Autodesk Fusion 360 part; units mm, degrees
note: some values were not read from the file. Chosen so that the rebuilt part matches the saved one: which face or edge a step refers to. Set by a fixed rule: which sketch regions a step uses.
(part 2 of 2)
  spline S262 degree 3 poles (19.3379, -14.9324) (18.8966, -14.9324) (18.4636, -14.9324) (18.0258, -14.9324) knots 0 0 0 0 1 1 1 1
  spline S263 degree 3 poles (18.0258, -14.9324) (18.0258, -13.8885) (18.0258, -12.8484) (18.0258, -11.8015) knots 0 0 0 0 1 1 1 1
  spline S264 degree 3 poles (18.0258, -11.8015) (18.3648, -11.8015) (18.7049, -11.8015) (19.0516, -11.8015) knots 0 0 0 0 1 1 1 1
  spline S265 degree 3 poles (19.0516, -11.8015) (19.0516, -10.138) (19.0516, -8.4811) (19.0516, -6.8195) knots 0 0 0 0 1 1 1 1
  spline S266 degree 3 poles (19.0516, -6.8195) (19.5983, -6.8195) (20.1384, -6.8195) (20.6851, -6.8195) knots 0 0 0 0 1 1 1 1
  spline S267 degree 3 poles (20.6851, -6.8195) (20.6851, -8.4753) (20.6851, -10.1322) (20.6851, -11.7957) knots 0 0 0 0 1 1 1 1
  spline S268 degree 3 poles (20.6851, -11.7957) (21.0317, -11.7957) (21.3719, -11.7957) (21.7168, -11.7957) knots 0 0 0 0 1 1 1 1
  spline S269 degree 3 poles (21.7168, -11.7957) (21.7168, -12.8425) (21.7168, -13.8827) (21.7168, -14.9324) knots 0 0 0 0 1 1 1 1
  spline S270 degree 3 poles (21.7168, -14.9324) (20.9273, -14.9324) (20.1368, -14.9324) (19.3379, -14.9324) knots 0 0 0 0 1 1 1 1
  spline S271 degree 3 poles (16.0875, -14.9324) (15.3573, -14.9324) (14.6354, -14.9324) (13.9087, -14.9324) knots 0 0 0 0 1 1 1 1
  spline S272 degree 3 poles (13.9087, -14.9324) (13.9087, -13.8886) (13.9087, -12.8484) (13.9087, -11.8016) knots 0 0 0 0 1 1 1 1
  spline S273 degree 3 poles (13.9087, -11.8016) (14.2476, -11.8016) (14.5877, -11.8016) (14.9344, -11.8016) knots 0 0 0 0 1 1 1 1
  spline S274 degree 3 poles (14.9344, -11.8016) (14.9344, -10.1381) (14.9344, -8.4812) (14.9344, -6.8195) knots 0 0 0 0 1 1 1 1
  spline S275 degree 3 poles (14.9344, -6.8195) (15.4811, -6.8195) (16.0212, -6.8195) (16.5679, -6.8195) knots 0 0 0 0 1 1 1 1
  spline S276 degree 3 poles (16.5679, -6.8195) (16.5679, -8.4752) (16.5679, -10.1321) (16.5679, -11.7956) knots 0 0 0 0 1 1 1 1
  spline S277 degree 3 poles (16.5679, -11.7956) (16.9145, -11.7956) (17.2547, -11.7956) (17.5996, -11.7956) knots 0 0 0 0 1 1 1 1
  spline S278 degree 3 poles (17.5996, -11.7956) (17.5996, -12.8425) (17.5996, -13.8826) (17.5996, -14.9324) knots 0 0 0 0 1 1 1 1
  spline S279 degree 3 poles (17.5996, -14.9324) (17.0991, -14.9324) (16.5975, -14.9324) (16.0875, -14.9324) knots 0 0 0 0 1 1 1 1
  spline S280 degree 3 poles (5.2528, -14.5323) (5.2528, -14.6681) (5.2528, -14.7955) (5.2528, -14.9276) knots 0 0 0 0 1 1 1 1
  spline S281 degree 3 poles (5.2528, -14.9276) (4.02, -14.9276) (2.7909, -14.9276) (1.5571, -14.9276) knots 0 0 0 0 1 1 1 1
  spline S282 degree 3 poles (1.5571, -14.9276) (1.5571, -13.8885) (1.5571, -12.8484) (1.5571, -11.8015) knots 0 0 0 0 1 1 1 1
  spline S283 degree 3 poles (1.5571, -11.8015) (1.8961, -11.8015) (2.2362, -11.8015) (2.5829, -11.8015) knots 0 0 0 0 1 1 1 1
  spline S284 degree 3 poles (2.5829, -11.8015) (2.5829, -10.138) (2.5829, -8.4811) (2.5829, -6.8195) knots 0 0 0 0 1 1 1 1
  spline S285 degree 3 poles (2.5829, -6.8195) (3.1296, -6.8195) (3.6697, -6.8195) (4.2164, -6.8195) knots 0 0 0 0 1 1 1 1
  spline S286 degree 3 poles (4.2164, -6.8195) (4.2164, -8.4753) (4.2164, -10.1322) (4.2164, -11.7957) knots 0 0 0 0 1 1 1 1
  spline S287 degree 3 poles (4.2164, -11.7957) (4.563, -11.7957) (4.9032, -11.7957) (5.2528, -11.7957) knots 0 0 0 0 1 1 1 1
  spline S288 degree 3 poles (5.2528, -11.7957) (5.2528, -12.7095) (5.2528, -13.6168) (5.2528, -14.5323) knots 0 0 0 0 1 1 1 1
  spline S289 degree 3 poles (19.0545, 0.9863) (19.0545, 1.7388) (19.0545, 2.4829) (19.0545, 3.2336) knots 0 0 0 0 1 1 1 1
  spline S290 degree 3 poles (19.0545, 3.2336) (18.7109, 3.2336) (18.3707, 3.2336) (18.0258, 3.2336) knots 0 0 0 0 1 1 1 1
  spline S291 degree 3 poles (18.0258, 3.2336) (18.0258, 4.2805) (18.0258, 5.3206) (18.0258, 6.3655) knots 0 0 0 0 1 1 1 1
  spline S292 degree 3 poles (18.0258, 6.3655) (19.2538, 6.3655) (20.4829, 6.3655) (21.7167, 6.3655) knots 0 0 0 0 1 1 1 1
  spline S293 degree 3 poles (21.7167, 6.3655) (21.7167, 5.3265) (21.7167, 4.2863) (21.7167, 3.2395) knots 0 0 0 0 1 1 1 1
  spline S294 degree 3 poles (21.7167, 3.2395) (21.3778, 3.2395) (21.0376, 3.2395) (20.6909, 3.2395) knots 0 0 0 0 1 1 1 1
  spline S295 degree 3 poles (20.6909, 3.2395) (20.6909, 1.576) (20.6909, -0.0809) (20.6909, -1.7426) knots 0 0 0 0 1 1 1 1
  spline S296 degree 3 poles (20.6909, -1.7426) (20.1443, -1.7426) (19.6042, -1.7426) (19.0545, -1.7426) knots 0 0 0 0 1 1 1 1
  spline S297 degree 3 poles (19.0545, -1.7426) (19.0545, -0.8365) (19.0545, 0.0708) (19.0545, 0.9863) knots 0 0 0 0 1 1 1 1
  spline S298 degree 3 poles (16.5709, -0.0972) (16.5709, -0.6496) (16.5709, -1.1937) (16.5709, -1.7426) knots 0 0 0 0 1 1 1 1
  spline S299 degree 3 poles (16.5709, -1.7426) (16.0271, -1.7426) (15.487, -1.7426) (14.9403, -1.7426) knots 0 0 0 0 1 1 1 1
  spline S300 degree 3 poles (14.9403, -1.7426) (14.9403, -0.0868) (14.9403, 1.5701) (14.9403, 3.2336) knots 0 0 0 0 1 1 1 1
  spline S301 degree 3 poles (14.9403, 3.2336) (14.5937, 3.2336) (14.2535, 3.2336) (13.9086, 3.2336) knots 0 0 0 0 1 1 1 1
  spline S302 degree 3 poles (13.9086, 3.2336) (13.9086, 4.2805) (13.9086, 5.3206) (13.9086, 6.3655) knots 0 0 0 0 1 1 1 1
  spline S303 degree 3 poles (13.9086, 6.3655) (15.1366, 6.3655) (16.3657, 6.3655) (17.5996, 6.3655) knots 0 0 0 0 1 1 1 1
  spline S304 degree 3 poles (17.5996, 6.3655) (17.5996, 5.3265) (17.5996, 4.2863) (17.5996, 3.2395) knots 0 0 0 0 1 1 1 1
  spline S305 degree 3 poles (17.5996, 3.2395) (17.2606, 3.2395) (16.9204, 3.2395) (16.5709, 3.2395) knots 0 0 0 0 1 1 1 1
  spline S306 degree 3 poles (16.5709, 3.2395) (16.5709, 2.1256) (16.5709, 1.0184) (16.5709, -0.0972) knots 0 0 0 0 1 1 1 1
  spline S307 degree 3 poles (19.8763, -5.7028) (19.5057, -6.0811) (19.0512, -6.2863) (18.5382, -6.3084) knots 0 0 0 0 1 1 1 1
  spline S308 degree 3 poles (18.5382, -6.3084) (17.8871, -6.3365) (17.2339, -6.3152) (16.5762, -6.3152) knots 0 0 0 0 1 1 1 1
  spline S309 degree 3 poles (16.5762, -6.3152) (16.5762, -4.9588) (16.5762, -3.5911) (16.5762, -2.2154) knots 0 0 0 0 1 1 1 1
  spline S310 degree 3 poles (16.5762, -2.2154) (16.5981, -2.2154) (16.6194, -2.2154) (16.6407, -2.2154) knots 0 0 0 0 1 1 1 1
  spline S311 degree 3 poles (16.6407, -2.2154) (17.1769, -2.2154) (17.713, -2.2138) (18.2492, -2.216) knots 0 0 0 0 1 1 1 1
  spline S312 degree 3 poles (18.2492, -2.216) (18.6308, -2.2175) (19.0001, -2.2829) (19.3445, -2.4547) knots 0 0 0 0 1 1 1 1
  spline S313 degree 3 poles (19.3445, -2.4547) (19.8492, -2.7066) (20.1823, -3.104) (20.3251, -3.6506) knots 0 0 0 0 1 1 1 1
  spline S314 degree 3 poles (20.3251, -3.6506) (20.4718, -4.2122) (20.439, -4.763) (20.1704, -5.2845) knots 0 0 0 0 1 1 1 1
  spline S315 degree 3 poles (20.1704, -5.2845) (20.0939, -5.4329) (19.9781, -5.561) (19.8763, -5.7028) knots 0 0 0 0 1 1 1 1
  spline S316 degree 3 poles (18.5377, -5.3752) (18.927, -5.274) (19.1788, -5.0271) (19.3006, -4.6473) knots 0 0 0 0 1 1 1 1
  spline S317 degree 3 poles (19.3006, -4.6473) (19.3662, -4.443) (19.3674, -4.2332) (19.3366, -4.0219) knots 0 0 0 0 1 1 1 1
  spline S318 degree 3 poles (19.3366, -4.0219) (19.265, -3.5312) (18.898, -3.1807) (18.4023, -3.1496) knots 0 0 0 0 1 1 1 1
  spline S319 degree 3 poles (18.4023, -3.1496) (18.1424, -3.1333) (17.881, -3.1411) (17.6203, -3.1384) knots 0 0 0 0 1 1 1 1
  spline S320 degree 3 poles (17.6203, -3.1384) (17.6161, -3.1384) (17.6118, -3.1449) (17.6084, -3.1476) knots 0 0 0 0 1 1 1 1
  spline S321 degree 3 poles (17.6084, -3.1476) (17.6084, -3.8994) (17.6084, -4.6506) (17.6084, -5.4225) knots 0 0 0 0 1 1 1 1
  spline S322 degree 3 poles (17.6084, -5.4225) (17.9168, -5.4076) (18.2205, -5.3929) (18.5377, -5.3752) knots 0 0 0 0 1 1 1 1
  spline S323 degree 3 poles (15.3406, -2.4936) (16.0423, -3.0161) (16.0475, -4.4321) (15.0414, -4.8191) knots 0 0 0 0 1 1 1 1
  spline S324 degree 3 poles (15.0414, -4.8191) (15.3108, -5.3205) (15.5798, -5.8213) (15.8523, -6.3286) knots 0 0 0 0 1 1 1 1
  spline S325 degree 3 poles (15.8523, -6.3286) (15.4534, -6.3286) (15.0653, -6.3286) (14.675, -6.3286) knots 0 0 0 0 1 1 1 1
  spline S326 degree 3 poles (14.675, -6.3286) (14.4647, -5.8864) (14.2534, -5.4444) (14.0449, -5.001) knots 0 0 0 0 1 1 1 1
  spline S327 degree 3 poles (14.0449, -5.001) (14.0209, -4.95) (13.9954, -4.9272) (13.9354, -4.9294) knots 0 0 0 0 1 1 1 1
  spline S328 degree 3 poles (13.9354, -4.9294) (13.7889, -4.9347) (13.6421, -4.9311) (13.4889, -4.9311) knots 0 0 0 0 1 1 1 1
  spline S329 degree 3 poles (13.4889, -4.9311) (13.4889, -5.3983) (13.4889, -5.8607) (13.4889, -6.3271) knots 0 0 0 0 1 1 1 1
  spline S330 degree 3 poles (13.4889, -6.3271) (13.1422, -6.3271) (12.8021, -6.3271) (12.4579, -6.3271) knots 0 0 0 0 1 1 1 1
  spline S331 degree 3 poles (12.4579, -6.3271) (12.4579, -4.9586) (12.4579, -3.5907) (12.4579, -2.2171) knots 0 0 0 0 1 1 1 1
  spline S332 degree 3 poles (12.4579, -2.2171) (12.479, -2.2161) (12.5003, -2.2142) (12.5215, -2.2142) knots 0 0 0 0 1 1 1 1
  spline S333 degree 3 poles (12.5215, -2.2142) (13.1604, -2.2141) (13.7992, -2.2129) (14.4381, -2.2146) knots 0 0 0 0 1 1 1 1
  spline S334 degree 3 poles (14.4381, -2.2146) (14.7645, -2.2155) (15.0702, -2.2889) (15.3406, -2.4936) knots 0 0 0 0 1 1 1 1
  spline S335 degree 3 poles (14.5491, -3.9706) (14.7482, -3.8541) (14.8308, -3.6559) (14.7702, -3.44) knots 0 0 0 0 1 1 1 1
  spline S336 degree 3 poles (14.7702, -3.44) (14.7198, -3.2602) (14.5592, -3.1252) (14.3613, -3.1158) knots 0 0 0 0 1 1 1 1
  spline S337 degree 3 poles (14.3613, -3.1158) (14.1508, -3.1058) (13.9397, -3.1102) (13.7288, -3.1087) knots 0 0 0 0 1 1 1 1
  spline S338 degree 3 poles (13.7288, -3.1087) (13.6496, -3.1082) (13.5705, -3.1087) (13.4928, -3.1087) knots 0 0 0 0 1 1 1 1
  spline S339 degree 3 poles (13.4928, -3.1087) (13.4928, -3.4221) (13.4928, -3.7256) (13.4928, -4.031) knots 0 0 0 0 1 1 1 1
  spline S340 degree 3 poles (13.4928, -4.031) (13.7592, -4.031) (14.02, -4.0354) (14.2806, -4.0285) knots 0 0 0 0 1 1 1 1
  spline S341 degree 3 poles (14.2806, -4.0285) (14.3669, -4.0263) (14.4525, -3.9952) (14.5491, -3.9706) knots 0 0 0 0 1 1 1 1
  spline S342 degree 3 poles (8.8148, -6.2867) (7.9838, -5.9726) (7.5385, -5.3685) (7.4511, -4.4994) knots 0 0 0 0 1 1 1 1
  spline S343 degree 3 poles (7.4511, -4.4994) (7.3936, -3.9287) (7.5204, -3.3995) (7.8763, -2.9414) knots 0 0 0 0 1 1 1 1
  spline S344 degree 3 poles (7.8763, -2.9414) (8.2477, -2.4633) (8.7507, -2.2206) (9.3469, -2.1623) knots 0 0 0 0 1 1 1 1
  spline S345 degree 3 poles (9.3469, -2.1623) (9.8261, -2.1155) (10.2832, -2.1946) (10.7025, -2.4367) knots 0 0 0 0 1 1 1 1
  spline S346 degree 3 poles (10.7025, -2.4367) (11.2593, -2.7583) (11.5798, -3.2502) (11.6844, -3.8784) knots 0 0 0 0 1 1 1 1
  spline S347 degree 3 poles (11.6844, -3.8784) (11.7777, -4.4385) (11.6991, -4.975) (11.3926, -5.4625) knots 0 0 0 0 1 1 1 1
  spline S348 degree 3 poles (11.3926, -5.4625) (11.0607, -5.9903) (10.5708, -6.2819) (9.9625, -6.3817) knots 0 0 0 0 1 1 1 1
  spline S349 degree 3 poles (9.9625, -6.3817) (9.5752, -6.4451) (9.1938, -6.4143) (8.8148, -6.2867) knots 0 0 0 0 1 1 1 1
  spline S350 degree 3 poles (9.7451, -5.4646) (10.0197, -5.4283) (10.2464, -5.3025) (10.4124, -5.0825) knots 0 0 0 0 1 1 1 1
  spline S351 degree 3 poles (10.4124, -5.0825) (10.6866, -4.7192) (10.7297, -4.3093) (10.616, -3.881) knots 0 0 0 0 1 1 1 1
  spline S352 degree 3 poles (10.616, -3.881) (10.4922, -3.415) (10.1205, -3.1151) (9.652, -3.0849) knots 0 0 0 0 1 1 1 1
  spline S353 degree 3 poles (9.652, -3.0849) (9.1837, -3.0546) (8.7796, -3.2983) (8.5947, -3.7278) knots 0 0 0 0 1 1 1 1
  spline S354 degree 3 poles (8.5947, -3.7278) (8.4712, -4.015) (8.4548, -4.3139) (8.5232, -4.6165) knots 0 0 0 0 1 1 1 1
  spline S355 degree 3 poles (8.5232, -4.6165) (8.6538, -5.1952) (9.1669, -5.5546) (9.7451, -5.4646) knots 0 0 0 0 1 1 1 1
  spline S356 degree 3 poles (4.7861, -3.7476) (5.0496, -3.7476) (5.3047, -3.7476) (5.5663, -3.7476) knots 0 0 0 0 1 1 1 1
  spline S357 degree 3 poles (5.5663, -3.7476) (5.5663, -3.2374) (5.5663, -2.7307) (5.5663, -2.219) knots 0 0 0 0 1 1 1 1
  spline S358 degree 3 poles (5.5663, -2.219) (5.9128, -2.219) (6.2529, -2.219) (6.598, -2.219) knots 0 0 0 0 1 1 1 1
  spline S359 degree 3 poles (6.598, -2.219) (6.598, -3.5851) (6.598, -4.9528) (6.598, -6.3259) knots 0 0 0 0 1 1 1 1
  spline S360 degree 3 poles (6.598, -6.3259) (6.2605, -6.3259) (5.9205, -6.3259) (5.5715, -6.3259) knots 0 0 0 0 1 1 1 1
  spline S361 degree 3 poles (5.5715, -6.3259) (5.5715, -5.7784) (5.5715, -5.2277) (5.5715, -4.6731) knots 0 0 0 0 1 1 1 1
  spline S362 degree 3 poles (5.5715, -4.6731) (5.0171, -4.6731) (4.4716, -4.6731) (3.9202, -4.6731) knots 0 0 0 0 1 1 1 1
  spline S363 degree 3 poles (3.9202, -4.6731) (3.9202, -5.2257) (3.9202, -5.7744) (3.9202, -6.3272) knots 0 0 0 0 1 1 1 1
  spline S364 degree 3 poles (3.9202, -6.3272) (3.5742, -6.3272) (3.2342, -6.3272) (2.89, -6.3272) knots 0 0 0 0 1 1 1 1
  spline S365 degree 3 poles (2.89, -6.3272) (2.89, -4.9586) (2.89, -3.5909) (2.89, -2.2187) knots 0 0 0 0 1 1 1 1
  spline S366 degree 3 poles (2.89, -2.2187) (3.23, -2.2187) (3.57, -2.2187) (3.9166, -2.2187) knots 0 0 0 0 1 1 1 1
  spline S367 degree 3 poles (3.9166, -2.2187) (3.9166, -2.7248) (3.9166, -3.2315) (3.9166, -3.7476) knots 0 0 0 0 1 1 1 1
  spline S368 degree 3 poles (3.9166, -3.7476) (4.2079, -3.7476) (4.4928, -3.7476) (4.7861, -3.7476) knots 0 0 0 0 1 1 1 1
  spline S369 degree 3 poles (22.9175, -6.4111) (22.3762, -6.4254) (21.8629, -6.3473) (21.4008, -6.0606) knots 0 0 0 0 1 1 1 1
  spline S370 degree 3 poles (21.4008, -6.0606) (21.263, -5.9751) (21.1384, -5.8684) (21.0063, -5.7703) knots 0 0 0 0 1 1 1 1
  spline S371 degree 3 poles (21.0063, -5.7703) (21.1969, -5.4911) (21.3764, -5.2281) (21.5574, -4.9629) knots 0 0 0 0 1 1 1 1
  spline S372 degree 3 poles (21.5574, -4.9629) (21.8467, -5.2515) (22.1842, -5.4301) (22.5817, -5.489) knots 0 0 0 0 1 1 1 1
  spline S373 degree 3 poles (22.5817, -5.489) (22.7472, -5.5135) (22.9146, -5.5251) (23.0774, -5.4773) knots 0 0 0 0 1 1 1 1
  spline S374 degree 3 poles (23.0774, -5.4773) (23.1505, -5.4558) (23.2248, -5.4235) (23.2856, -5.3785) knots 0 0 0 0 1 1 1 1
  spline S375 degree 3 poles (23.2856, -5.3785) (23.4555, -5.2526) (23.4475, -5.0356) (23.2715, -4.9181) knots 0 0 0 0 1 1 1 1
  spline S376 degree 3 poles (23.2715, -4.9181) (23.1088, -4.8095) (22.9173, -4.7803) (22.7327, -4.7317) knots 0 0 0 0 1 1 1 1
  spline S377 degree 3 poles (22.7327, -4.7317) (22.4467, -4.6562) (22.1557, -4.5935) (21.8784, -4.4933) knots 0 0 0 0 1 1 1 1
  spline S378 degree 3 poles (21.8784, -4.4933) (21.5626, -4.3793) (21.3157, -4.1722) (21.2023, -3.8388) knots 0 0 0 0 1 1 1 1
  spline S379 degree 3 poles (21.2023, -3.8388) (20.9904, -3.2162) (21.2975, -2.5667) (21.9309, -2.2991) knots 0 0 0 0 1 1 1 1
  spline S380 degree 3 poles (21.9309, -2.2991) (22.2119, -2.1804) (22.5074, -2.14) (22.8099, -2.1493) knots 0 0 0 0 1 1 1 1
  spline S381 degree 3 poles (22.8099, -2.1493) (23.3266, -2.1652) (23.8053, -2.3004) (24.2246, -2.6141) knots 0 0 0 0 1 1 1 1
  spline S382 degree 3 poles (24.2246, -2.6141) (24.269, -2.6472) (24.3112, -2.6833) (24.3582, -2.7211) knots 0 0 0 0 1 1 1 1
  spline S383 degree 3 poles (24.3582, -2.7211) (24.1702, -2.9751) (23.9841, -3.2265) (23.7958, -3.481) knots 0 0 0 0 1 1 1 1
  spline S384 degree 3 poles (23.7958, -3.481) (23.5573, -3.2871) (23.2915, -3.1547) (22.9932, -3.0916) knots 0 0 0 0 1 1 1 1
  spline S385 degree 3 poles (22.9932, -3.0916) (22.81, -3.0529) (22.6254, -3.0318) (22.4411, -3.0831) knots 0 0 0 0 1 1 1 1
  spline S386 degree 3 poles (22.4411, -3.0831) (22.3965, -3.0955) (22.3516, -3.1151) (22.3135, -3.1412) knots 0 0 0 0 1 1 1 1
  spline S387 degree 3 poles (22.3135, -3.1412) (22.1419, -3.2588) (22.1442, -3.5034) (22.3312, -3.5903) knots 0 0 0 0 1 1 1 1
  spline S388 degree 3 poles (22.3312, -3.5903) (22.4872, -3.6628) (22.6594, -3.7048) (22.8281, -3.7446) knots 0 0 0 0 1 1 1 1
  spline S389 degree 3 poles (22.8281, -3.7446) (23.1543, -3.8216) (23.4844, -3.8837) (23.789, -4.0313) knots 0 0 0 0 1 1 1 1
  spline S390 degree 3 poles (23.789, -4.0313) (24.0819, -4.1733) (24.316, -4.3737) (24.4065, -4.7003) knots 0 0 0 0 1 1 1 1
  spline S391 degree 3 poles (24.4065, -4.7003) (24.5516, -5.2235) (24.4064, -6.0124) (23.5524, -6.2929) knots 0 0 0 0 1 1 1 1
  spline S392 degree 3 poles (23.5524, -6.2929) (23.3522, -6.3587) (23.1349, -6.3728) (22.9175, -6.4111) knots 0 0 0 0 1 1 1 1
  spline S393 degree 3 poles (-1.7096, -4.7079) (-1.7861, -4.2326) (-1.7511, -3.7755) (-1.5499, -3.342) knots 0 0 0 0 1 1 1 1
  spline S394 degree 3 poles (-1.5499, -3.342) (-1.2408, -2.6758) (-0.7062, -2.3015) (0.0089, -2.1814) knots 0 0 0 0 1 1 1 1
  spline S395 degree 3 poles (0.0089, -2.1814) (0.4535, -2.1068) (0.889, -2.1471) (1.2998, -2.3478) knots 0 0 0 0 1 1 1 1
  spline S396 degree 3 poles (1.2998, -2.3478) (1.6948, -2.5408) (1.9652, -2.8548) (2.1625, -3.252) knots 0 0 0 0 1 1 1 1
  spline S397 degree 3 poles (2.1625, -3.252) (1.8658, -3.397) (1.5737, -3.5398) (1.2783, -3.6842) knots 0 0 0 0 1 1 1 1
  spline S398 degree 3 poles (1.2783, -3.6842) (1.1567, -3.415) (0.9617, -3.2273) (0.6845, -3.1336) knots 0 0 0 0 1 1 1 1
  spline S399 degree 3 poles (0.6845, -3.1336) (0.2351, -2.9817) (-0.2715, -3.1751) (-0.5172, -3.6064) knots 0 0 0 0 1 1 1 1
  spline S400 degree 3 poles (-0.5172, -3.6064) (-0.7704, -4.0506) (-0.7716, -4.5093) (-0.5183, -4.9527) knots 0 0 0 0 1 1 1 1
  spline S401 degree 3 poles (-0.5183, -4.9527) (-0.3165, -5.3059) (0.0047, -5.4883) (0.4124, -5.4753) knots 0 0 0 0 1 1 1 1
  spline S402 degree 3 poles (0.4124, -5.4753) (0.8181, -5.4624) (1.1014, -5.2458) (1.28, -4.8789) knots 0 0 0 0 1 1 1 1
  spline S403 degree 3 poles (1.28, -4.8789) (1.5722, -5.0215) (1.8643, -5.1642) (2.1626, -5.3099) knots 0 0 0 0 1 1 1 1
  spline S404 degree 3 poles (2.1626, -5.3099) (1.915, -5.8044) (1.5549, -6.1614) (1.0233, -6.3208) knots 0 0 0 0 1 1 1 1
  spline S405 degree 3 poles (1.0233, -6.3208) (0.2175, -6.5625) (-0.7701, -6.3349) (-1.3208, -5.6058) knots 0 0 0 0 1 1 1 1
  spline S406 degree 3 poles (-1.3208, -5.6058) (-1.5217, -5.3399) (-1.6474, -5.0416) (-1.7096, -4.7079) knots 0 0 0 0 1 1 1 1
  spline S407 degree 3 poles (18.5309, -5.3767) (18.2205, -5.3929) (17.9168, -5.4076) (17.6084, -5.4225) knots 0 0 0 0 1 1 1 1
  spline S408 degree 3 poles (17.6084, -5.4225) (17.6084, -4.6506) (17.6084, -3.8994) (17.6084, -3.1476) knots 0 0 0 0 1 1 1 1
  spline S409 degree 3 poles (17.6084, -3.1476) (17.6118, -3.1449) (17.6161, -3.1384) (17.6203, -3.1384) knots 0 0 0 0 1 1 1 1
  spline S410 degree 3 poles (17.6203, -3.1384) (17.881, -3.1411) (18.1424, -3.1333) (18.4023, -3.1496) knots 0 0 0 0 1 1 1 1
  spline S411 degree 3 poles (18.4023, -3.1496) (18.898, -3.1807) (19.265, -3.5312) (19.3366, -4.0219) knots 0 0 0 0 1 1 1 1
  spline S412 degree 3 poles (19.3366, -4.0219) (19.3674, -4.2332) (19.3662, -4.443) (19.3006, -4.6473) knots 0 0 0 0 1 1 1 1
  spline S413 degree 3 poles (19.3006, -4.6473) (19.1788, -5.0271) (18.927, -5.274) (18.5309, -5.3767) knots 0 0 0 0 1 1 1 1
  spline S414 degree 3 poles (14.5438, -3.974) (14.4525, -3.9952) (14.3669, -4.0263) (14.2806, -4.0285) knots 0 0 0 0 1 1 1 1
  spline S415 degree 3 poles (14.2806, -4.0285) (14.02, -4.0354) (13.7592, -4.031) (13.4928, -4.031) knots 0 0 0 0 1 1 1 1
  spline S416 degree 3 poles (13.4928, -4.031) (13.4928, -3.7256) (13.4928, -3.4221) (13.4928, -3.1087) knots 0 0 0 0 1 1 1 1
  spline S417 degree 3 poles (13.4928, -3.1087) (13.5705, -3.1087) (13.6496, -3.1082) (13.7288, -3.1087) knots 0 0 0 0 1 1 1 1
  spline S418 degree 3 poles (13.7288, -3.1087) (13.9397, -3.1102) (14.1508, -3.1058) (14.3613, -3.1158) knots 0 0 0 0 1 1 1 1
  spline S419 degree 3 poles (14.3613, -3.1158) (14.5592, -3.1252) (14.7198, -3.2602) (14.7702, -3.44) knots 0 0 0 0 1 1 1 1
  spline S420 degree 3 poles (14.7702, -3.44) (14.8308, -3.6559) (14.7482, -3.8541) (14.5438, -3.974) knots 0 0 0 0 1 1 1 1
  spline S421 degree 3 poles (9.7378, -5.4657) (9.1669, -5.5546) (8.6538, -5.1952) (8.5232, -4.6165) knots 0 0 0 0 1 1 1 1
  spline S422 degree 3 poles (8.5232, -4.6165) (8.4548, -4.3139) (8.4712, -4.015) (8.5947, -3.7278) knots 0 0 0 0 1 1 1 1
  spline S423 degree 3 poles (8.5947, -3.7278) (8.7796, -3.2983) (9.1837, -3.0546) (9.652, -3.0849) knots 0 0 0 0 1 1 1 1
  spline S424 degree 3 poles (9.652, -3.0849) (10.1205, -3.1151) (10.4922, -3.415) (10.616, -3.881) knots 0 0 0 0 1 1 1 1
  spline S425 degree 3 poles (10.616, -3.881) (10.7297, -4.3093) (10.6866, -4.7192) (10.4124, -5.0825) knots 0 0 0 0 1 1 1 1
  spline S426 degree 3 poles (10.4124, -5.0825) (10.2464, -5.3025) (10.0197, -5.4283) (9.7378, -5.4657) knots 0 0 0 0 1 1 1 1
  line L22 (0.9434, 11.6) -> (1.2, 11.6)
  line L23 (21.4434, 39.6) -> (21.7, 39.6)
  line L24 (-21.7, 39.6) -> (-21.4434, 39.6)
  line L25 (19.3, 11.6) -> (19.5566, 11.6)
  line L26 (-21.7, 11.6) -> (-21.4434, 11.6)
  line L27 (-1.2, 39.6) -> (-0.9434, 39.6)
  line L28 (-15, 63.5) -> (15, 63.5) construction
  line L29 (11, 66.555) -> (-11, 66.555)
  line L30 (-11, 66.555) -> (-11, 60.445)
  line L31 (-11, 60.445) -> (11, 60.445)
  line L32 (11, 60.445) -> (11, 66.555)
  line L33 (11, 66.555) -> (-11, 60.445) construction
  line L34 (-11, 66.555) -> (11, 60.445) construction
  arc A8 (0.9434, 11.6) -> (-0.9434, 11.6) centre (0, 16) ccw
  line L35 (-1.2, 11.6) -> (-0.9434, 11.6)
  circle A9 centre (23.0823, -36.9623) radius 4.15
  circle A10 centre (-7.547, -36.9993) radius 4.15
  arc A11 (-19.5566, 39.6) -> (-21.4434, 39.6) centre (-20.5, 44) ccw
  line L36 (-19.5566, 39.6) -> (-19.3, 39.6)
  arc A12 (21.4434, 11.6) -> (19.5566, 11.6) centre (20.5, 16) ccw
  line L37 (21.4434, 11.6) -> (21.7, 11.6)
  arc A13 (21.4434, 39.6) -> (19.5566, 39.6) centre (20.5, 44) ccw
  line L38 (19.3, 39.6) -> (19.5566, 39.6)
  arc A14 (-19.5566, 11.6) -> (-21.4434, 11.6) centre (-20.5, 16) ccw
  line L39 (-19.5566, 11.6) -> (-19.3, 11.6)
  arc A15 (0.9434, 39.6) -> (-0.9434, 39.6) centre (0, 44) ccw
  line L40 (0.9434, 39.6) -> (1.2, 39.6)
  point P0 (0, 63.5)
  dimension "d156" = 22
  dimension "d157" = 6.11
  constraint coincident A2.centre L28.start
  constraint coincident A0.centre L28.end
  constraint horizontal L29
  constraint perpendicular L29 L30
  constraint parallel L29 L31
  constraint parallel L30 L32
  constraint coincident L33 P0
  constraint coincident L34 P0
  constraint midpoint L28 P0
  measures "d156" distance of L30.end L31.end
  measures "d157" distance of L29.end L30.end
extrude "Extrude11" cut sketch "Sketch6" against normal blind 0.4 contours S0 S1 S2 S3 S4 | S316 S317 S318 S319 S320 S321 S322 S407 S408 S409 S410 S411 S412 S413 | S335 S336 S337 S338 S339 S340 S341 S414 S415 S416 S417 S418 S419 S420 | S350 S351 S352 S353 S354 S355 S421 S422 S423 S424 S425 S426
extrude "Extrude12" add sketch "Sketch5" against normal blind 1 from surface at -2 contours L0 L2 L3 L23 L24 L25 L26 | L0 L1 L2 L19 L21 L22
chamfer "Chamfer3" distance 1 angle 45 2 edges at (0, 58.5, 0) (0, -50, 0)
extrude "Extrude13" cut sketch "Sketch6" against normal blind 0.4 from surface at 1 contours L29 L30 L31 L32
extrude "Extrude14" cut sketch "Sketch2" along normal blind 7 contours A31 | A32
equation "d1 = 60 mm - 0.2 mm"
equation "d157 = 4.11 mm + 2 mm"
